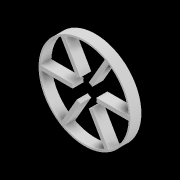
# Autodesk Inventor part: Spol_rotor_parameteriserad_03 [2020-11-22]
Saved by Autodesk Inventor 2020 (Build 240168000, 168)
## iProperties
Created: 2020-11-22
Part Number: Spol_rotor_parameteriserad_03 [2020-11-22]
Material: Generic
Document SubType Name: Modeling
Designer: Gottfrid
Density: 1 g/cm^3
Appearance: Default
Author: Gottfrid
Autodesk Inventor part; units mm, degrees
ref_plane "YZ Plane" through (0, 0, 0) normal (1, 0, 0) x (0, 1, 0)
ref_plane "XZ Plane" through (0, 0, 0) normal (0, 1, 0) x (-1, 0, 0)
ref_plane "XY Plane" through (0, 0, 0) normal (0, 0, 1) x (1, 0, 0)
sketch "Sketch1" plane through (0, 0, 0) normal (0, 0, 1) x (1, 0, 0)
  circle A0 centre (0, 0) radius 42.5
  circle A1 centre (0, 0) radius 41
  circle A2 centre (0, 0) radius 11.25
  line L0 (11.1051, 1.8) -> (40.9605, 1.8)
  line L1 (42.5, 0) -> (43.6334, 0) construction
  line L2 (-59.7267, 0) -> (60.8601, 0) projected
  line L3 (11.1051, -1.8) -> (40.9605, -1.8)
  line L4 (3.9937, 10.5173) -> (18.9214, 36.3728)
  line L5 (7.1114, 8.7173) -> (22.0391, 34.5728)
  line L6 (-7.1114, 8.7173) -> (-22.0391, 34.5728)
  line L7 (-3.9937, 10.5173) -> (-18.9214, 36.3728)
  line L8 (-11.1051, -1.8) -> (-40.9605, -1.8)
  line L9 (-11.1051, 1.8) -> (-40.9605, 1.8)
  line L10 (-3.9937, -10.5173) -> (-18.9214, -36.3728)
  line L11 (-7.1114, -8.7173) -> (-22.0391, -34.5728)
  line L12 (7.1114, -8.7173) -> (22.0391, -34.5728)
  line L13 (3.9937, -10.5173) -> (18.9214, -36.3728)
  point P0 (11.1051, -1.8)
  point P1 (22.0391, -34.5728)
  point P2 (7.1114, -8.7173)
  point P3 (3.9937, -10.5173)
  point P4 (18.9214, -36.3728)
  point P5 (-3.9937, -10.5173)
  point P6 (-7.1114, -8.7173)
  point P7 (-11.1051, -1.8)
  point P8 (-11.1051, 1.8)
  point P9 (-7.1114, 8.7173)
  point P10 (-3.9937, 10.5173)
  point P11 (3.9937, 10.5173)
  dimension "d0" = 85
  dimension "d1" = 82
  dimension "d2" = 22.5
  dimension "d3" = 1.8
  dimension "d6" = 360
  constraints: 26 end point, 3 coincident, 2 horizontal, 2 symmetric about line, 1 horizontal alignment, 45 other
  measures "d3" distance between parallel lines of L0 L2
extrude "Extrusion1" add sketch "Sketch1" along normal blind 10 contours L2 A1 A0 | A0 L2 A1 | L2 A2 L0 A1 | A1 L3 A2 L2 | L2 A2 L8 A1 | A1 L9 A2 L2 | L5 A2 L4 A1 | A1 L13 A2 L12 | A1 L7 A2 L6 | L11 A2 L10 A1
equation "\"d0\" = D_yttreSpolRotor"
equation "\"d1\" = D_yttreSpolRotor - d_yttreRing"
equation "\"d2\" = 2 * r_yttre + d_yttreRing_1"
equation "\"d3\" = d_stöttor"
equation "\"d8\" = h_spolRotor"
equation "\"D_yttreSpolRotor\" = 85"
equation "\"h_spolRotor\" = h_rullager"
equation "\"d_yttreRing\" = 3"
equation "\"r_yttre\" = 10"
equation "\"d_yttreRing_1\" = 2.5"
equation "\"d_stöttor\" = 1.8"
equation "\"h_rullager\" = 10"
body "Solid1"
